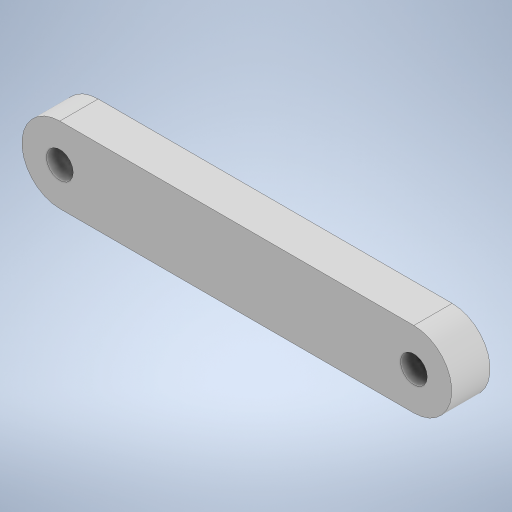
# Autodesk Inventor part: ArmOuter
Saved by Autodesk Inventor 2023 (Build 270158000, 158)
## iProperties
Created: 2023-06-03
Part Number: ArmOuter
Material: Ogólny
Document SubType Name: Modeling
Designer: Kamil
Density: 1 g/cm^3
Appearance: Domyślna
Author: Kamil
Autodesk Inventor part; units mm, degrees
ref_plane "YZ Plane" through (0, 0, 0) normal (1, 0, 0) x (0, 1, 0)
ref_plane "XZ Plane" through (0, 0, 0) normal (0, 1, 0) x (-1, 0, 0)
ref_plane "XY Plane" through (0, 0, 0) normal (0, 0, 1) x (1, 0, 0)
sketch "Szkic1" plane through (0, 0, 0) normal (0, 0, 1) x (1, 0, 0)
  line L0 (46.2, 9.8993) -> (0, 9.9005)
  circle A0 centre (46.2019, 4.9521) radius 4.9472
  line L1 (0, 0) -> (46.2, 0.005)
  circle A1 centre (0.0001, 4.9503) radius 4.9503
  circle A2 centre (0.0001, 4.9503) radius 1.75
  circle A3 centre (18.487, 4.9458) radius 1.75
  circle A4 centre (46.2021, 4.9479) radius 1.75
  point P0 (0, 0)
  point P1 (-4.95, 0)
  point P2 (0.0003, 9.9005)
  point P3 (0.0007, 0)
  dimension "d0" = 3.5
  dimension "d1" = 3.5
  dimension "d2" = 3.5
  constraints: 5 centre point, 4 end point, 4 tangent, 1 coincident, 2 other
  measures "d0" diameter of A2
  measures "d1" diameter of A3
  measures "d2" diameter of A4
extrude "Wyciągnięcie proste1" add sketch "Szkic1" along normal blind 5
sketch "Szkic3" plane through (0, 0, 5) normal (0, 0, 1) x (1, 0, 0)
  circle A0 centre (18.487, 4.9458) radius 1.75 projected
  point P0 (0, 0)
extrude "Wyciągnięcie proste3" add sketch "Szkic3" against normal up to surface (5 mm away)
